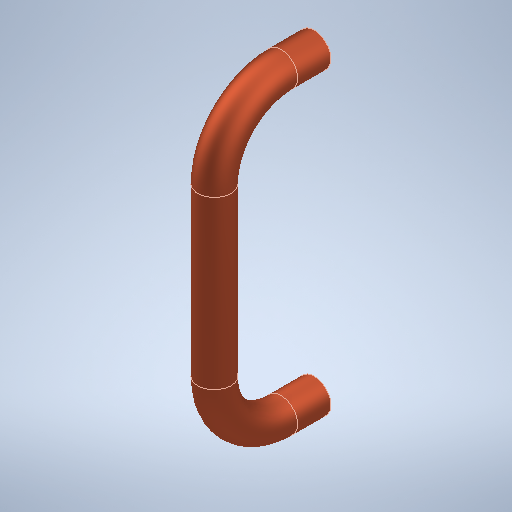
# Autodesk Inventor part: front_frame_support
Saved by Autodesk Inventor 2025.2 (Build 292293000, 293)
## iProperties
Created: 2025-08-03
Part Number: front_frame_support
Material: Copper, Alloy
Document SubType Name: Modeling
Designer: chris
Density: 8.92 g/cm^3
Appearance: Copper - Satin
Author: chris
Autodesk Inventor part; units mm, degrees
ref_plane "YZ Plane" through (0, 0, 0) normal (1, 0, 0) x (0, 1, 0)
ref_plane "XZ Plane" through (0, 0, 0) normal (0, 1, 0) x (-1, 0, 0)
ref_plane "XY Plane" through (0, 0, 0) normal (0, 0, 1) x (1, 0, 0)
sketch "Sketch1" plane through (0, 0, 0) normal (0, 1, 0) x (-1, 0, 0)
  circle A0 centre (0, 0) radius 2.5
  dimension "d0" = 5
  constraints: 1 centre point, 1 coincident
  measures "d0" diameter of A0
extrude "Extrusion1" add sketch "Sketch1" along normal blind 25
sketch "Sketch3" plane through (0, 25, 0) normal (0, 1, 0) x (1, 0, 0)
  circle A0 centre (0, 0) radius 2.5
  line L0 (-5.8989, 10) -> (6.7654, 10)
  dimension "d4" = 5
  dimension "d5" = 20
  constraints: 2 end point, 1 centre point, 1 coincident, 1 horizontal
  measures "d4" diameter of A0
  measures "d5" diameter of point (0, 0) L0
revolve "Revolution1" add sketch "Sketch3" angle 90 about axis through (-5.8989, 25, -10) along (-1, 0, 0)
sketch "Sketch4" plane through (0, 0, 0) normal (0, -1, 0) x (1, 0, 0)
  circle A0 centre (0, 0) radius 2.5
  line L0 (10.1723, -10) -> (-10.0505, -10)
  dimension "d7" = 5
  dimension "d8" = 20
  constraints: 2 end point, 1 centre point, 1 coincident, 1 horizontal
  measures "d7" diameter of A0
  measures "d8" diameter of point (0, 0) L0
revolve "Revolution2" add sketch "Sketch4" angle 90 about axis through (10.1723, 0, -10) along (1, 0, 0)
sketch "Sketch5" plane through (0, -10, -10) normal (0, 0, -1) x (-1, 0, 0)
  circle A0 centre (0, 0) radius 2.5
  circle A1 centre (0, 0) radius 2.5 projected
  circle A2 centre (0, 45) radius 2.5
  circle A3 centre (0, 45) radius 2.5 projected
  point P0 (0, 10)
  dimension "d10" = 5
  dimension "d11" = 5
  constraints: 2 centre point, 2 concentric
  measures "d10" diameter of A0
  measures "d11" diameter of A2
extrude "Extrusion2" add sketch "Sketch5" along normal blind 5
sketch "Sketch6" plane through (0, 35, -15) normal (0, 0, -1) x (-1, 0, 0)
  circle A0 centre (0, 0) radius 2.5
  circle A1 centre (0, 0) radius 2.5 projected
  circle A2 centre (0, -45) radius 2.5
  circle A3 centre (0, -45) radius 2.5 projected
  point P0 (0, -35)
  dimension "d14" = 5
  dimension "d15" = 5
  constraints: 2 centre point, 2 concentric
  measures "d14" diameter of A0
  measures "d15" diameter of A2
hole "Hole1" at (0, 35, -15) at (0, -10, -15) direction (0, 0, 1) diameter 3.1 depth 5 tip angle 118
thread "Thread1" size "M3x0.5" class "6H" standard "ANSI Metric M Profile" full length
thread "Thread2" size "M3x0.5" class "6H" standard "ANSI Metric M Profile" full length
body "Solid1"
